Autodesk Fusion 360 part; units mm, degrees
(part 2 of 2)
sketch "Sketch21 (3)" plane through (0, 0, 1) normal (0, 0, 1) x (-1, 0, 0) in component "2"
  circle A0 centre (-8.5, 0) radius 9.5
  arc A1 (-18.8, -6.8) -> (-15.3, -10.3) centre (-15.3, -6.8) ccw
  line L0 (-18.8, -6.8) -> (-18.8, 6.8)
  arc A2 (-15.3, 10.3) -> (-18.8, 6.8) centre (-15.3, 6.8) ccw
  line L1 (-15.3, 10.3) -> (21, 10.3)
  line L2 (21, 10.3) -> (21, -10.3)
  line L3 (21, -10.3) -> (-15.3, -10.3)
  line L4 (1.8, -10.3) -> (1.8, 10.3)
  line L5 (0, 0) -> (-18.8, 0) construction
  arc A3 (-21, -7.5) -> (-17.5, -11) centre (-17.5, -7.5) ccw
  line L6 (-17.5, -11) -> (17.5, -11)
  arc A4 (17.5, -11) -> (21, -7.5) centre (17.5, -7.5) ccw
  line L7 (21, -7.5) -> (21, 7.5)
  arc A5 (21, 7.5) -> (17.5, 11) centre (17.5, 7.5) ccw
  line L8 (17.5, 11) -> (-17.5, 11)
  arc A6 (-17.5, 11) -> (-21, 7.5) centre (-17.5, 7.5) ccw
  line L9 (-21, 7.5) -> (-21, -7.5)
  circle A7 centre (-8, 0) radius 6.5
  circle A8 centre (12.6, 0) radius 6.5
  dimension "d400_1" = 19
  dimension "d401_1" = 20.6
  constraint coincident L3 L4.start
  constraint coincident L1 L4.end
  constraint perpendicular L1 L4
  constraint coincident L5.start origin
  constraint midpoint L0 L5.end
  constraint coincident A0.centre L5
  measures "d400_1" diameter of A0
  measures "d401_1" distance of L0 L4
fillet "Fillet10'" radius 3.5 8 edges at (21, -11, 0) (21, 11, 0) (-21, 11, 0) (-21, -11, 0) (19, -9, 1) (19, 9, 1) (-19, 9, 1) (-19, -9, 1) on bodies 2 in component "1"
sketch "Sketch18 (4)" plane through (-21, 0, 0) normal (-1, 0, 0) x (0, -1, 0) in component "1"
  line L0 (7.5, -3) -> (7.5, 3)
  line L1 (7.5, 3) -> (-7.5, 3)
  line L2 (-7.5, 3) -> (-7.5, -3)
  line L3 (-7.5, -3) -> (7.5, -3)
  line L4 (6, 3) -> (-6, 3)
  line L5 (-6, 3) -> (-6, 0)
  line L6 (-6, 0) -> (6, 0)
  line L7 (6, 0) -> (6, 3)
  line L8 (6, 3) -> (-6, 0) construction
  line L9 (-6, 3) -> (6, 0) construction
  line L10 (0, -3) -> (0, 3)
  point P0 (0, 1.5)
  dimension "d458" = 12
  dimension "d459" = 3
  constraint horizontal L4
  constraint perpendicular L4 L5
  constraint parallel L4 L6
  constraint parallel L5 L7
  constraint coincident L1 L4.start
  constraint coincident L8 P0
  constraint coincident L9 P0
  constraint midpoint L3 L10.start
  constraint midpoint L4 L10.end
  constraint vertical L10
  measures "d458" distance of L5.end L6.end
  measures "d459" distance of L4.start L6.end
extrude "Extrude17'" cut sketch "Sketch18 (4)" against normal blind 2.7 contours L1 L4 L6 L7 L10 | L1 L4 L5 L6 L10 bodies 2 in component "1"
sketch "Sketch19" plane through (0, 11, 0) normal (0, 1, 0) x (-1, 0, 0) in component "1"
  line L0 (17.5, -3) -> (17.5, 3)
  line L1 (17.5, 3) -> (-17.5, 3)
  line L2 (-17.5, 3) -> (-17.5, -3)
  line L3 (-17.5, -3) -> (17.5, -3)
  line L4 (-17.5, 0) -> (-16.9461, 0)
  line L5 (-16.9461, 0) -> (17.5, 0)
  point P0 (-12, 0)
  point P1 (12, 0)
  dimension "d462" = 12
  dimension "d463" = 12
  constraint midpoint L2 L4.start
  constraint perpendicular L2 L4
  constraint midpoint L0 L5.end
  constraint perpendicular L0 L5
  constraint coincident L5 P0
  constraint coincident L5 P1
  measures "d462" distance of origin P0
  measures "d463" distance of origin P1
hole "Hole2'" at (12, 11, 0) at (-12, 11, 0) direction (0, -1, 0) diameter 2.529 depth 2 tip angle 118 bodies 2 in component "1"
thread "Thread1" "ISO Metric profile 3.0 M3x0.5 6H" in component "1"
mirror "Mirror1" about plane through (0, 0, 0) normal (0, 1, 0) of "Hole2'" in component "1"
sketch "Sketch1 (10)" plane through (0, 0, 0) normal (0, 0, 1) x (1, 0, 0) in component "Resistance Paer"
  line L0 (17, 9) -> (-17, 9)
  line L1 (-17, 9) -> (-17, -9)
  line L2 (-17, -9) -> (17, -9)
  line L3 (17, -9) -> (17, 9)
  line L4 (17, 9) -> (-17, -9) construction
  line L5 (-17, 9) -> (17, -9) construction
  dimension "d138_1" = 18
  dimension "d139_1" = 34
  constraint horizontal L0
  constraint perpendicular L0 L1
  constraint parallel L0 L2
  constraint parallel L1 L3
  constraint coincident L4 origin
  constraint coincident L5 origin
  measures "d138_1" distance of L0.start L2.end
  measures "d139_1" distance of L0.start L0.end
extrude "Extrude1''''''''''''''" add sketch "Sketch1 (10)" along normal blind 0.06 separate body makes body 17 in component "Resistance Paer"
sketch "Sketch1 (11)" plane through (0, 0, 0) normal (0, 0, -1) x (1, 0, 0) in component "nylon wire vertical"
  line L0 (17, -9) -> (17, 9) construction
  line L1 (17, 9) -> (-17, 9) construction
  line L2 (-17, 9) -> (-17, -9)
  line L3 (-17, -9) -> (17, -9) construction
  line L4 (15, 8) -> (-15, 8) construction
  line L5 (-15, 8) -> (-15, -8) construction
  line L6 (-15, -8) -> (15, -8) construction
  line L7 (15, -8) -> (15, 8) construction
  line L8 (15, 8) -> (-15, -8) construction
  line L9 (-15, 8) -> (15, -8) construction
  line L10 (15, 8) -> (-15, 8)
  line L11 (-15, 8) -> (-15, 3)
  line L12 (-15, 3) -> (15, 3)
  line L13 (15, 3) -> (15, 8)
  line L14 (15, 8) -> (-15, 3) construction
  line L15 (-15, 8) -> (15, 3) construction
  line L16 (15, -8) -> (-15, -8)
  line L17 (-15, -8) -> (-15, -3)
  line L18 (-15, -3) -> (15, -3)
  line L19 (15, -3) -> (15, -8)
  line L20 (15, -8) -> (-15, -3) construction
  line L21 (-15, -8) -> (15, -3) construction
  point P0 (0, 5.5)
  point P1 (0, -5.5)
  dimension "d151_1" = 5
  dimension "d153_1" = 2
  dimension "d172_1" = 6
  constraint horizontal L4
  constraint perpendicular L4 L5
  constraint parallel L4 L6
  constraint parallel L5 L7
  constraint coincident L8 origin
  constraint coincident L9 origin
  constraint horizontal L10
  constraint perpendicular L10 L11
  constraint parallel L10 L12
  constraint parallel L11 L13
  constraint coincident L14 P0
  constraint coincident L15 P0
  constraint horizontal L16
  constraint perpendicular L16 L17
  constraint parallel L16 L18
  constraint parallel L17 L19
  constraint coincident L20 P1
  constraint coincident L21 P1
  constraint equal L11 L17
  constraint coincident L5 L11.end
  measures "d151_1" distance of L4.end L11.end
  measures "d153_1" distance of L2 L5
  measures "d172_1" distance of L12 L18
extrude "Extrude1'''''''''''''''" add sketch "Sketch1 (11)" along normal blind 0.2 separate body makes body 18 at (5, -4.6667, 0) makes body 19 at (5, 4.6667, 0) in component "nylon wire vertical"
move_face "OffsetFaces1" offset 3 2 faces at (15, 6.3333, -0.1333) (15, -6.3333, -0.1333) on bodies 18 19 in component "nylon wire vertical"
sketch "Sketch2 (4)" plane through (0, 0, 0) normal (0, 0, 1) x (-1, 0, 0) in component "nylon wire vertical"
  line L0 (-18, 8) -> (-18, 3)
  line L1 (-18, 3) -> (15, 3)
  line L2 (15, 3) -> (15, 8)
  line L3 (15, 8) -> (-18, 8)
  line L4 (-18, -8) -> (-17.8, -8)
  line L5 (-17.8, -8) -> (-17.8, -3)
  line L6 (-17.8, -3) -> (-18, -3)
  line L7 (-18, -3) -> (-18, -8)
  line L8 (-18, -8) -> (-17.8, -3) construction
  line L9 (-17.8, -8) -> (-18, -3) construction
  line L10 (-18, 3) -> (-17.8, 3)
  line L11 (-17.8, 3) -> (-17.8, 8)
  line L12 (-17.8, 8) -> (-18, 8)
  line L13 (-18, 8) -> (-18, 3)
  line L14 (-18, 3) -> (-17.8, 8) construction
  line L15 (-17.8, 3) -> (-18, 8) construction
  point P0 (-17.9, -5.5)
  point P1 (-17.9, 5.5)
  point P2 (-18, -8)
  point P3 (-18, -3)
  dimension "d157_1" = 0.2
  constraint horizontal L4
  constraint perpendicular L4 L5
  constraint parallel L4 L6
  constraint parallel L5 L7
  constraint coincident L8 P0
  constraint coincident L9 P0
  constraint horizontal L10
  constraint perpendicular L10 L11
  constraint parallel L10 L12
  constraint parallel L11 L13
  constraint coincident L0.end L1.start
  constraint coincident L14 P1
  constraint coincident L15 P1
  constraint coincident P2 L4.start
  constraint coincident P3 L6.end
  constraint coincident L0.start L3.end
  constraint equal L6 L10
  measures "d157_1" distance of L11.end L0.start
extrude "Extrude2''''" add sketch "Sketch2 (4)" along normal blind 8 contours L0 L1 L3 L10 L11 L12 L13 | L4 L5 L6 L7 bodies 18 19 in component "nylon wire vertical"
sketch "Sketch1 (12)" plane through (0, 0, 0) normal (0, 0, -1) x (1, 0, 0) in component "termistor (2)"
  line L0 (17, -9) -> (17, 9)
  line L1 (17, 9) -> (-17, 9)
  line L2 (-17, 9) -> (-17, -9)
  line L3 (-17, -9) -> (17, -9)
  line L4 (-2.5, 2.5) -> (18, 2.5)
  line L5 (18, 2.5) -> (18, -2.5)
  line L6 (18, -2.5) -> (-2.5, -2.5)
  line L7 (-2.5, -2.5) -> (-2.5, 2.5)
  line L8 (-2.5, 2.5) -> (18, -2.5) construction
  line L9 (18, 2.5) -> (-2.5, -2.5) construction
  line L10 (18, 3) -> (18, 8)
  line L11 (0, 0) -> (7.75, 0) construction
  line L12 (-2.5, -8) -> (-2.5, 8)
  point P0 (7.75, 0)
  dimension "d160_2" = 5
  constraint horizontal L4
  constraint perpendicular L4 L5
  constraint parallel L4 L6
  constraint parallel L5 L7
  constraint coincident L8 P0
  constraint coincident L9 P0
  constraint coincident L4.end L10
  constraint coincident L11.start origin
  constraint horizontal L11
  constraint coincident P0 L11.end
  constraint coincident L4.start L12
  measures "d160_2" distance of L4.start L6.end
extrude "Extrude1''''''''''''''''" add sketch "Sketch1 (12)" along normal blind 0.2 separate body contours L0 L4 L6 L7 L12 | L0 L4 L5 L6 makes body 20 in component "termistor (2)"
sketch "Sketch2 (5)" plane through (0, 0, 0) normal (0, 0, 1) x (-1, 0, 0) in component "termistor (2)"
  line L0 (-18, 2.5) -> (-18, -2.5)
  line L1 (-18, -2.5) -> (2.5, -2.5)
  line L2 (2.5, -2.5) -> (2.5, 2.5)
  line L3 (2.5, 2.5) -> (-18, 2.5)
  line L4 (-18, -2.5) -> (-17.8, -2.5)
  line L5 (-17.8, -2.5) -> (-17.8, 2.5)
  line L6 (-17.8, 2.5) -> (-18, 2.5)
  line L7 (-18, 2.5) -> (-18, -2.5)
  line L8 (-18, -2.5) -> (-17.8, 2.5) construction
  line L9 (-17.8, -2.5) -> (-18, 2.5) construction
  line L10 (-18, -0.9562) -> (-17.8, -0.9562)
  line L11 (-17.8, -0.9562) -> (-17.8, 0.9562)
  line L12 (-17.8, 0.9562) -> (-18, 0.9562)
  line L13 (-18, 0.9562) -> (-18, -0.9562)
  line L14 (-18, -0.9562) -> (-17.8, 0.9562) construction
  line L15 (-17.8, -0.9562) -> (-18, 0.9562) construction
  point P0 (-17.9, 0)
  point P1 (-17.9, 0)
  dimension "d163_2" = 0.2
  constraint horizontal L4
  constraint perpendicular L4 L5
  constraint parallel L4 L6
  constraint parallel L5 L7
  constraint coincident L0.end L1.start
  constraint coincident L8 P1
  constraint coincident L9 P1
  constraint coincident L0.start L3.end
  constraint horizontal L10
  constraint perpendicular L10 L11
  constraint parallel L10 L12
  constraint parallel L11 L13
  constraint coincident L7 L10.start
  constraint coincident L14 P1
  constraint coincident L15 P1
  constraint coincident P1 P0
  measures "d163_2" distance of L5.end L0.start
extrude "Extrude2'''''" add sketch "Sketch2 (5)" along normal blind 7 contours L0 L3 L5 L6 L7 L12 | L0 L1 L4 L5 L7 L10 bodies 20 in component "termistor (2)"
sketch "Sketch1 (13)" plane through (0, 0, 0) normal (0, 0, 1) x (1, 0, 0) in component "silicon membrane"
  line L0 (19, 10.5) -> (-19, 10.5)
  line L1 (-19, 10.5) -> (-19, -10.5)
  line L2 (-19, -10.5) -> (19, -10.5)
  line L3 (19, -10.5) -> (19, 10.5)
  line L4 (19, 10.5) -> (-19, -10.5) construction
  line L5 (-19, 10.5) -> (19, -10.5) construction
  dimension "d166_1" = 21
  dimension "d167_1" = 38
  constraint horizontal L0
  constraint perpendicular L0 L1
  constraint parallel L0 L2
  constraint parallel L1 L3
  constraint coincident L4 origin
  constraint coincident L5 origin
  measures "d166_1" distance of L0.start L2.end
  measures "d167_1" distance of L0.start L0.end
extrude "Extrude1'''''''''''''''''" add sketch "Sketch1 (13)" along normal mid plane 3.5 separate body makes body 21 in component "silicon membrane"
fillet "Fillet1" radius 3.5 4 edges at (-19, 10.5, 0) (-19, -10.5, 0) (19, -10.5, 0) (19, 10.5, 0) on bodies 21 in component "silicon membrane"
sketch "Sketch4 (2)" plane through (0, 0, 1.75) normal (0, 0, 1) x (-1, 0, 0) in component "Silicon Tactile  (2)"
  arc A0 (-19, -7) -> (-15.5, -10.5) centre (-15.5, -7) ccw
  line L0 (-15.5, -10.5) -> (15.5, -10.5)
  arc A1 (15.5, -10.5) -> (19, -7) centre (15.5, -7) ccw
  line L1 (19, -7) -> (19, 7)
  arc A2 (19, 7) -> (15.5, 10.5) centre (15.5, 7) ccw
  line L2 (15.5, 10.5) -> (-15.5, 10.5)
  arc A3 (-15.5, 10.5) -> (-19, 7) centre (-15.5, 7) ccw
  line L3 (-19, 7) -> (-19, -7)
  line L4 (0, 0) -> (0, 7.8)
  line L5 (0, 0) -> (-17.8, 0)
  line L6 (-18, 8) -> (-18, 3)
  line L7 (-18, 3) -> (-17.8, 3)
  line L8 (-17.8, 3) -> (-17.8, 8)
  line L9 (-17.8, 8) -> (-18, 8)
  line L10 (-17.8, 2.5) -> (-18, 2.5)
  line L11 (-18, 2.5) -> (-18, 0.9562)
  line L12 (-18, 0.9562) -> (-17.8, 0.9562)
  line L13 (-17.8, 0.9562) -> (-17.8, 2.5)
  line L14 (-18, -2.5) -> (-17.8, -2.5)
  line L15 (-17.8, -2.5) -> (-17.8, -0.9562)
  line L16 (-17.8, -0.9562) -> (-18, -0.9562)
  line L17 (-18, -0.9562) -> (-18, -2.5)
  line L18 (-18, -3) -> (-18, -8)
  line L19 (-18, -8) -> (-17.8, -8)
  line L20 (-17.8, -8) -> (-17.8, -3)
  line L21 (-17.8, -3) -> (-18, -3)
  line L22 (-13.5, 7.8) -> (-8.5, 7.8)
  line L23 (-8.5, 7.8) -> (-8.5, 8)
  line L24 (-8.5, 8) -> (-13.5, 8)
  line L25 (-13.5, 8) -> (-13.5, 7.8)
  line L26 (-2.5, 7.8) -> (2.5, 7.8)
  line L27 (2.5, 7.8) -> (2.5, 8)
  line L28 (2.5, 8) -> (-2.5, 8)
  line L29 (-2.5, 8) -> (-2.5, 7.8)
  line L30 (8.5, 7.8) -> (13.5, 7.8)
  line L31 (13.5, 7.8) -> (13.5, 8)
  line L32 (13.5, 8) -> (8.5, 8)
  line L33 (8.5, 8) -> (8.5, 7.8)
  line L34 (13.65, 8.15) -> (8.35, 8.15)
  line L35 (8.35, 8.15) -> (8.35, 7.65)
  line L36 (8.35, 7.65) -> (13.65, 7.65)
  line L37 (13.65, 7.65) -> (13.65, 8.15)
  line L38 (2.65, 8.15) -> (-2.65, 8.15)
  line L39 (-2.65, 8.15) -> (-2.65, 7.65)
  line L40 (-2.65, 7.65) -> (2.65, 7.65)
  line L41 (2.65, 7.65) -> (2.65, 8.15)
  line L42 (-8.35, 8.15) -> (-13.65, 8.15)
  line L43 (-13.65, 8.15) -> (-13.65, 7.65)
  line L44 (-13.65, 7.65) -> (-8.35, 7.65)
  line L45 (-8.35, 7.65) -> (-8.35, 8.15)
  line L46 (-18.15, 8.15) -> (-18.15, 2.85)
  line L47 (-18.15, 2.85) -> (-17.65, 2.85)
  line L48 (-17.65, 2.85) -> (-17.65, 8.15)
  line L49 (-17.65, 8.15) -> (-18.15, 8.15)
  line L50 (-18.15, 2.65) -> (-18.15, 0.8062)
  line L51 (-18.15, 0.8062) -> (-17.65, 0.8062)
  line L52 (-17.65, 0.8062) -> (-17.65, 2.65)
  line L53 (-17.65, 2.65) -> (-18.15, 2.65)
  line L54 (-18.15, -0.8062) -> (-18.15, -2.65)
  line L55 (-18.15, -2.65) -> (-17.65, -2.65)
  line L56 (-17.65, -2.65) -> (-17.65, -0.8062)
  line L57 (-17.65, -0.8062) -> (-18.15, -0.8062)
  line L58 (-18.15, -2.85) -> (-18.15, -8.15)
  line L59 (-18.15, -8.15) -> (-17.65, -8.15)
  line L60 (-17.65, -8.15) -> (-17.65, -2.85)
  line L61 (-17.65, -2.85) -> (-18.15, -2.85)
  dimension "d177_1" = 0.15
  dimension "d178_1" = 0.15
  dimension "d179_1" = 0.15
  dimension "d180_1" = 0.15
  dimension "d181_1" = 0.15
  dimension "d182_1" = 0.15
  dimension "d183_1" = 0.15
  constraint coincident L4.start L5.start
  constraint vertical L4
  constraint perpendicular L4 L5
  constraint midpoint L4.end L26
  constraint coincident L5.end L15
sketch "Sketch17 (3)" plane through (0, 0, 0) normal (0, 0, 1) x (1, 0, 0) in component "4"
  line L0 (21.5, 11.5) -> (-21.5, 11.5)
  line L1 (-21.5, 11.5) -> (-21.5, -11.5)
  line L2 (-21.5, -11.5) -> (21.5, -11.5)
  line L3 (21.5, -11.5) -> (21.5, 11.5)
  line L4 (21.5, 11.5) -> (-21.5, -11.5) construction
  line L5 (-21.5, 11.5) -> (21.5, -11.5) construction
  line L6 (-23.75, -13.75) -> (23.75, -13.75)
  line L7 (23.75, -13.75) -> (23.75, 13.75)
  line L8 (23.75, 13.75) -> (-23.75, 13.75)
  line L9 (-23.75, 13.75) -> (-23.75, -13.75)
  dimension "d1_1_1_1" = 43
  dimension "d2_1_1_1" = 23
  dimension "d3_1_1_1" = 2.25
  constraint horizontal L0
  constraint perpendicular L0 L1
  constraint parallel L0 L2
  constraint parallel L1 L3
  constraint coincident L4 origin
  constraint coincident L5 origin
  measures "d1_1_1_1" distance of L0.start L0.end
  measures "d2_1_1_1" distance of L0.start L2.end
extrude "Extrude17''" add sketch "Sketch17 (3)" against normal blind 14 separate body makes body 22 in component "4"
sketch "Sketch29" plane through (0, 0, 1) normal (0, 0, 1) x (-1, 0, 0) in component "2"
  circle A0 centre (12.6, 0) radius 3.5
  circle A1 centre (12.6, 0) radius 4.5
sketch "Sketch30" plane through (21, 0, 0) normal (1, 0, 0) x (0, 1, 0) in component "2"
  line L0 (7.5, -1) -> (7.5, 1)
  line L1 (7.5, 1) -> (-7.5, 1)
  line L2 (-7.5, 1) -> (-7.5, -1)
  line L3 (-7.5, -1) -> (7.5, -1)
  line L4 (0, 0) -> (0, -1)
  line L5 (6, -1) -> (-6, -1)
  line L6 (-6, -1) -> (-6, 1.5539)
  line L7 (-6, 1.5539) -> (6, 1.5539)
  line L8 (6, 1.5539) -> (6, -1)
  line L9 (6, -1) -> (-6, 1.5539) construction
  line L10 (-6, -1) -> (6, 1.5539) construction
  point P0 (0, 0.277)
  dimension "d485" = 12
  constraint coincident L4.start origin
  constraint midpoint L3 L4.end
  constraint horizontal L5
  constraint perpendicular L5 L6
  constraint parallel L5 L7
  constraint parallel L6 L8
  constraint coincident L3 L5.start
  constraint coincident L9 P0
  constraint coincident L10 P0
  constraint coincident L4 P0
  measures "d485" distance of L6.end L7.end
extrude "Extrude34" cut sketch "Sketch30" against normal blind 7 contours L1 L3 L5 L6 L8 | L1 L6 L7 L8 bodies 16 in component "2"
sketch "Sketch18 (5)" plane through (0, 0, -3) normal (0, 0, -1) x (1, 0, 0) in component "3"
  arc A0 (-17.5, 11) -> (-21, 7.5) centre (-17.5, 7.5) ccw
  line L0 (-21, 7.5) -> (-21, -7.5)
  arc A1 (-21, -7.5) -> (-17.5, -11) centre (-17.5, -7.5) ccw
  line L1 (-17.5, -11) -> (17.5, -11)
  arc A2 (17.5, -11) -> (21, -7.5) centre (17.5, -7.5) ccw
  line L2 (21, -7.5) -> (21, 7.5)
  arc A3 (21, 7.5) -> (17.5, 11) centre (17.5, 7.5) ccw
  line L3 (17.5, 11) -> (-17.5, 11) construction
  line L4 (-21, 0) -> (21, 0) construction
  circle A4 centre (-12.6, 0) radius 5.5 construction
  circle A5 centre (12.6, 0) radius 5.5 construction
  circle A6 centre (-12.6, 0) radius 6.5
  circle A7 centre (-12.6, 0) radius 4.5
  circle A8 centre (12.6, 0) radius 6.5
  circle A9 centre (12.6, 0) radius 4
  line L5 (-15, 5) -> (-15, -5)
  line L6 (-15, -5) -> (-19, -5)
  line L7 (-19, -5) -> (-19, 5)
  line L8 (-19, 5) -> (-15, 5)
  dimension "d491" = 11
  dimension "d492" = 8.4
  dimension "d493" = 8.4
  dimension "d494" = 1
  dimension "d495" = -1
  dimension "d496" = 1
  dimension "d497" = -1.5
  constraint midpoint L0 L4.start
  constraint midpoint L2 L4.end
  constraint coincident L4 A4.centre
  constraint coincident L4 A5.centre
  constraint equal A4 A5
  measures "d491" diameter of A4
  measures "d492" distance of L4.start A4.centre
  measures "d493" distance of L4.end A5.centre
extrude "Extrude19" cut sketch "Sketch18 (5)" against normal blind 2 contours A6 A7 L5 L6 L8 | A6 A7 L5 L6 L7 L8 | A6 L7 | A8 bodies 15 in component "3"
sketch "Sketch19 (2)" plane through (0, 0, -3) normal (0, 0, -1) x (1, 0, 0) in component "3"
  circle A0 centre (12.6, 0) radius 4
  circle A1 centre (12.6, 0) radius 2.75
  dimension "d500" = 5.5
  constraint concentric A0 A1
  measures "d500" diameter of A1
fillet "Fillet13" radius 3.5 8 edges at (21.5, 11.5, -7) (-21.5, 11.5, -7) (-21.5, -11.5, -7) (21.5, -11.5, -7) (-23.75, 13.75, -7) (23.75, 13.75, -7) (23.75, -13.75, -7) (-23.75, -13.75, -7) on bodies 22 in component "4"
sketch "Sketch19 (3)" plane through (0, -13.75, 0) normal (0, -1, 0) x (1, 0, 0) in component "4"
  line L0 (-20.25, 0) -> (-20.25, -14)
  line L1 (-20.25, -14) -> (20.25, -14)
  line L2 (20.25, -14) -> (20.25, 0)
  line L3 (20.25, 0) -> (-20.25, 0)
  line L4 (-20.25, -3) -> (20.25, -3)
  line L5 (-20.25, -11) -> (20.25, -11)
  point P0 (-12, -3)
  point P1 (12, -3)
  point P2 (-12, -11)
  point P3 (12, -11)
  dimension "d505" = 12
  dimension "d506" = 3
  dimension "d507" = 3
  dimension "d508" = 12
  dimension "d509" = 12
  dimension "d510" = 12
  constraint coincident L0 L4.start
  constraint coincident L2 L4.end
  constraint perpendicular L2 L4
  constraint coincident L4 P0
  constraint coincident L4 P1
  constraint coincident L0 L5.start
  constraint coincident L2 L5.end
  constraint perpendicular L2 L5
  constraint coincident L5 P2
  constraint coincident L5 P3
  measures "d505" horizontal distance of origin P0
  measures "d506" distance of L3 L4
  measures "d507" distance of L1 L5
  measures "d508" horizontal distance of origin P2
  measures "d509" horizontal distance of origin P3
  measures "d510" horizontal distance of origin P1
hole "Hole1" at (-12, -13.75, -3) at (-12, -13.75, -11) at (12, -13.75, -3) at (12, -13.75, -11) direction (0, 1, 0) diameter 2.529 depth 45 tip angle 118 bodies 22 in component "4"
thread "Thread1'" "ISO Metric profile 3.0 M3x0.5 6H" in component "4"
sketch "Sketch20 (4)" plane through (0, 13.75, 0) normal (0, 1, 0) x (-1, 0, 0) in component "4"
  circle A0 centre (-12, -3) radius 1.2645
  circle A1 centre (12, -3) radius 1.2645
  circle A2 centre (12, -11) radius 1.2645
  circle A3 centre (-12, -11) radius 1.2645
  line L0 (-20.25, 0) -> (-20.25, -14)
  line L1 (-20.25, -14) -> (20.25, -14)
  line L2 (20.25, -14) -> (20.25, 0)
  line L3 (20.25, 0) -> (-20.25, 0)
  line L4 (-3, -11) -> (-3, -3)
  arc A4 (-3, -3) -> (-5, -3) centre (-4, -3) ccw
  line L5 (-5, -3) -> (-5, -11)
  arc A5 (-5, -11) -> (-3, -11) centre (-4, -11) ccw
  line L6 (-4, -11) -> (-4, -3) construction
  line L7 (0, 0) -> (0, -14) construction
  line L8 (4, 0) -> (4, -14) construction
  line L9 (-4, -14) -> (-4, 0) construction
  line L10 (3, -11) -> (3, -3)
  line L11 (5, -3) -> (5, -11)
  arc A6 (5, -3) -> (3, -3) centre (4, -3) ccw
  arc A7 (3, -11) -> (5, -11) centre (4, -11) ccw
  point P0 (-4, -7)
  dimension "d524" = 2
  dimension "d525" = 8
  dimension "d562" = 4
  dimension "d564" = 4
  dimension "d565" = 3
  constraint tangent L4 A4
  constraint tangent A4 L5
  constraint parallel L4 L5
  constraint tangent L5 A5
  constraint tangent L4 A5
  constraint coincident L6 P0
  constraint midpoint L6 P0
  constraint coincident L7.start origin
  constraint midpoint L1 L7.end
  constraint coincident L3 L8.start
  constraint coincident L1 L8.end
  constraint perpendicular L1 L8
  constraint coincident L1 L9.start
  constraint coincident L3 L9.end
  constraint perpendicular L3 L9
  constraint coincident P0 L9
  constraint coincident A4.centre L9
  constraint symmetric L4.start L7 L10.start
  constraint symmetric L4.end L7 L10.end
  constraint symmetric A4.end L7 L11.start
  constraint symmetric L5.end L7 L11.end
  constraint symmetric A4 L7 A6
  constraint symmetric A5 L7 A7
  measures "d524" distance of L4 L5
  measures "d525" distance of A4.end L5.end
  measures "d562" distance of A4.centre L7
  measures "d564" distance of L7 L8
  measures "d565" distance of L3 A6.centre
extrude "Extrude21" cut sketch "Sketch20 (4)" against normal blind 27.5 contours L4 A4 L5 A5 | L10 L11 A6 A7 bodies 22 in component "4"
sketch "Sketch31" plane through (0, 0, 1) normal (0, 0, 1) x (-1, 0, 0) in component "2"
  line L0 (-14, -6) -> (-21, -6)
  line L1 (-21, -6) -> (-21, -7.5)
  arc A0 (-21, -7.5) -> (-17.5, -11) centre (-17.5, -7.5) ccw
  line L2 (-17.5, -11) -> (17.5, -11)
  arc A1 (17.5, -11) -> (21, -7.5) centre (17.5, -7.5) ccw
  line L3 (21, -7.5) -> (21, 7.5)
  arc A2 (21, 7.5) -> (17.5, 11) centre (17.5, 7.5) ccw
  line L4 (17.5, 11) -> (-17.5, 11)
  arc A3 (-17.5, 11) -> (-21, 7.5) centre (-17.5, 7.5) ccw
  line L5 (-21, 7.5) -> (-21, 6)
  line L6 (-21, 6) -> (-14, 6)
  arc A4 (-14, -2.5) -> (-14, 2.5) centre (-8, 0) ccw
  circle A5 centre (12.6, 0) radius 6.5
  spline S0 degree 5 poles (0, -11) (0, -10.12) (0, -8.36) (0, -5.72) (0, -2.2) (0, 2.2) (0, 5.72) (0, 8.36) (0, 10.12) (0, 11) knots 0 0 0 0 0 0 0.2 0.4 0.6 0.8 1 1 1 1 1 1
  line L7 (-7.5, -8) -> (7.5, -8)
  line L8 (7.5, -8) -> (7.5, -14)
  line L9 (7.5, -14) -> (-7.5, -14)
  line L10 (-7.5, -14) -> (-7.5, -8)
  line L11 (-7.5, -8) -> (7.5, -14) construction
  line L12 (7.5, -8) -> (-7.5, -14) construction
  line L13 (-7.5, 8) -> (7.5, 8)
  line L14 (7.5, 8) -> (7.5, 14)
  line L15 (7.5, 14) -> (-7.5, 14)
  line L16 (-7.5, 14) -> (-7.5, 8)
  line L17 (-7.5, 8) -> (7.5, 14) construction
  line L18 (7.5, 8) -> (-7.5, 14) construction
  line L19 (-14, 6) -> (-14, 2.5)
  line L20 (-14, -2.5) -> (-14, -6)
  point P0 (0, -11)
  point P1 (0, 11)
  dimension "d528" = 6
  dimension "d529" = 6
  dimension "d530" = 15
  dimension "d531" = 15
  constraint midpoint L2 P0
  constraint midpoint L4 P1
  constraint horizontal L7
  constraint perpendicular L7 L8
  constraint parallel L7 L9
  constraint parallel L8 L10
  constraint coincident L11 P0
  constraint coincident L12 P0
  constraint coincident P0 S0.start
  constraint horizontal L13
  constraint perpendicular L13 L14
  constraint parallel L13 L15
  constraint parallel L14 L16
  constraint coincident L17 P1
  constraint coincident L18 P1
  constraint coincident P1 S0.end
  measures "d528" distance of L13.start L15.end
  measures "d529" distance of L7.start L9.end
  measures "d530" distance of L8.end L9.end
  measures "d531" distance of L13.start L13.end
extrude "Extrude35" cut sketch "Sketch31" against normal blind 2 contours L2 S0 L7 L10 | L2 S0 L7 L8 | L4 S0 L13 L16 | L4 S0 L13 L14 bodies 16 in component "2"
sketch "Sketch20 (5)" plane through (0, 0, 3) normal (0, 0, 1) x (-1, 0, 0) in component "1"
  line L0 (21, -6) -> (18.9641, -6)
  arc A0 (15.5, -9) -> (18.9641, -6) centre (15.5, -5.5) ccw
  line L1 (15.5, -9) -> (-15.5, -9)
  arc A1 (-19, -5.5) -> (-15.5, -9) centre (-15.5, -5.5) ccw
  line L2 (-19, -5.5) -> (-19, 5.5)
  arc A2 (-15.5, 9) -> (-19, 5.5) centre (-15.5, 5.5) ccw
  line L3 (-15.5, 9) -> (15.5, 9)
  arc A3 (18.9641, 6) -> (15.5, 9) centre (15.5, 5.5) ccw
  line L4 (18.9641, 6) -> (21, 6)
  line L5 (21, 6) -> (21, 7.5)
  arc A4 (21, 7.5) -> (17.5, 11) centre (17.5, 7.5) ccw
  line L6 (17.5, 11) -> (-17.5, 11)
  arc A5 (-17.5, 11) -> (-21, 7.5) centre (-17.5, 7.5) ccw
  line L7 (-21, 7.5) -> (-21, -7.5)
  arc A6 (-21, -7.5) -> (-17.5, -11) centre (-17.5, -7.5) ccw
  line L8 (-17.5, -11) -> (17.5, -11)
  arc A7 (17.5, -11) -> (21, -7.5) centre (17.5, -7.5) ccw
  line L9 (21, -7.5) -> (21, -6)
  line L10 (0, -11) -> (0, 11)
  line L11 (-7.5, -8) -> (7.5, -8)
  line L12 (7.5, -8) -> (7.5, -14)
  line L13 (7.5, -14) -> (-7.5, -14)
  line L14 (-7.5, -14) -> (-7.5, -8)
  line L15 (-7.5, -8) -> (7.5, -14) construction
  line L16 (7.5, -8) -> (-7.5, -14) construction
  line L17 (-7.5, 8) -> (7.5, 8)
  line L18 (7.5, 8) -> (7.5, 14)
  line L19 (7.5, 14) -> (-7.5, 14)
  line L20 (-7.5, 14) -> (-7.5, 8)
  line L21 (-7.5, 8) -> (7.5, 14) construction
  line L22 (7.5, 8) -> (-7.5, 14) construction
  point P0 (0, -11)
  point P1 (0, 11)
  dimension "d534" = 15
  dimension "d535" = 6
  dimension "d536" = 6
  dimension "d537" = 15
  constraint midpoint L8 P0
  constraint midpoint L6 P1
  constraint horizontal L11
  constraint perpendicular L11 L12
  constraint parallel L11 L13
  constraint parallel L12 L14
  constraint coincident L15 P0
  constraint coincident L16 P0
  constraint coincident P0 L10.start
  constraint horizontal L17
  constraint perpendicular L17 L18
  constraint parallel L17 L19
  constraint parallel L18 L20
  constraint coincident L21 P1
  constraint coincident L22 P1
  constraint coincident P1 L10.end
  measures "d534" distance of L12.end L13.end
  measures "d535" distance of L11.start L13.end
  measures "d536" distance of L17.start L19.end
  measures "d537" distance of L18.end L19.end
extrude "Extrude18''" cut sketch "Sketch20 (5)" against normal blind 6 contours L1 L8 L10 L12 | L1 L10 L11 L12 | L1 L8 L10 L14 | L1 L10 L11 L14 | L3 L10 L17 L20 | L3 L10 L17 L18 | L3 L6 L10 L18 | L3 L6 L10 L20 bodies 2 in component "1"
sketch "Sketch20 (6)" plane through (0, 0, -3) normal (0, 0, -1) x (1, 0, 0) in component "3"
  circle A0 centre (12.6, 0) radius 6.5
  arc A1 (-16.7533, -5) -> (-16.7533, 5) centre (-12.6, 0) ccw
  line L0 (-16.7533, -5) -> (-19, -5)
  line L1 (-19, -5) -> (-19, -1.1358)
  arc A2 (-19, 1.1358) -> (-19, -1.1358) centre (-12.6, 0) ccw
  line L2 (-19, 1.1358) -> (-19, 5)
  line L3 (-19, 5) -> (-16.7533, 5)
  arc A3 (-17.5, 11) -> (-21, 7.5) centre (-17.5, 7.5) ccw
  line L4 (-21, 7.5) -> (-21, -7.5)
  arc A4 (-21, -7.5) -> (-17.5, -11) centre (-17.5, -7.5) ccw
  line L5 (-17.5, -11) -> (17.5, -11)
  arc A5 (17.5, -11) -> (21, -7.5) centre (17.5, -7.5) ccw
  line L6 (21, -7.5) -> (21, 7.5)
  arc A6 (21, 7.5) -> (17.5, 11) centre (17.5, 7.5) ccw
  line L7 (17.5, 11) -> (-17.5, 11)
  spline S0 degree 5 poles (0, 11) (0, 10.12) (0, 8.36) (0, 5.72) (0, 2.2) (0, -2.2) (0, -5.72) (0, -8.36) (0, -10.12) (0, -11) knots 0 0 0 0 0 0 0.2 0.4 0.6 0.8 1 1 1 1 1 1
  line L8 (6, 11) -> (-6, 11)
  line L9 (-6, 11) -> (-6, 8.5)
  line L10 (-6, 8.5) -> (6, 8.5)
  line L11 (6, 8.5) -> (6, 11)
  line L12 (6, 11) -> (-6, 8.5) construction
  line L13 (-6, 11) -> (6, 8.5) construction
  line L14 (6, -11) -> (-6, -11)
  line L15 (-6, -11) -> (-6, -8.5)
  line L16 (-6, -8.5) -> (6, -8.5)
  line L17 (6, -8.5) -> (6, -11)
  line L18 (6, -11) -> (-6, -8.5) construction
  line L19 (-6, -11) -> (6, -8.5) construction
  point P0 (0, 9.75)
  point P1 (0, -9.75)
  dimension "d540" = 12
  dimension "d541" = 12
  dimension "d542" = 2.5
  dimension "d543" = 2.5
  constraint midpoint L7 S0.start
  constraint midpoint L5 S0.end
  constraint horizontal L8
  constraint perpendicular L8 L9
  constraint parallel L8 L10
  constraint parallel L9 L11
  constraint coincident L7 L8.start
  constraint coincident L12 P0
  constraint coincident L13 P0
  constraint coincident S0 P0
  constraint horizontal L14
  constraint perpendicular L14 L15
  constraint parallel L14 L16
  constraint parallel L15 L17
  constraint coincident L5 L14.start
  constraint coincident L18 P1
  constraint coincident L19 P1
  constraint coincident S0 P1
  measures "d540" distance of L9.end L10.end
  measures "d541" distance of L15.end L16.end
  measures "d542" distance of L14.start L16.end
  measures "d543" distance of L8.start L10.end
extrude "Extrude21'" add sketch "Sketch20 (6)" along normal blind 3 contours L7 S0 L8 L9 L10 | L7 S0 L8 L10 L11 | L5 S0 L14 L15 L16 | L5 S0 L14 L16 L17 bodies 15 in component "3"
sketch "Sketch21 (4)" plane through (0, -11, 0) normal (0, -1, 0) x (1, 0, 0) in component "3"
  line L0 (-17.5, 3) -> (-17.5, -3)
  line L1 (-17.5, -3) -> (-6, -3)
  line L2 (-6, -3) -> (-6, -6)
  line L3 (6, -6) -> (6, -3)
  line L4 (6, -3) -> (17.5, -3)
  line L5 (17.5, -3) -> (17.5, 3)
  line L6 (17.5, 3) -> (-17.5, 3)
  line L7 (6, -6) -> (6, -3)
  line L8 (-6, -3) -> (-6, -6)
  line L9 (0, 0) -> (0, -4.9341) construction
  line L10 (-4, -4) -> (4, -4)
  line L11 (6, -6) -> (-6, -6)
  point P0 (0, -4)
  dimension "d560" = 8
  dimension "d561" = 2
  constraint parallel L7 L8
  constraint coincident L3.start L7.start
  constraint coincident L2.end L8.end
  constraint coincident L4 L3.end
  constraint coincident L9.start origin
  constraint perpendicular L6 L9
  constraint horizontal L10
  constraint midpoint L10 P0
  constraint coincident L9 P0
  measures "d560" distance of L10.start L10.end
  measures "d561" distance of L10 L11
hole "Hole1'" at (-4, -11, -4) at (4, -11, -4) direction (0, 1, 0) diameter 2 depth 45 tip angle 118 bodies 15 in component "3"
sketch "Sketch21 (5)" plane through (-23.75, 0, 0) normal (-1, 0, 0) x (0, -1, 0) in component "4"
  line L0 (10.25, -14) -> (10.25, 0)
  line L1 (10.25, 0) -> (-10.25, 0)
  line L2 (-10.25, 0) -> (-10.25, -14)
  line L3 (-10.25, -14) -> (10.25, -14)
  line L4 (0, 0) -> (0, -14) construction
  line L5 (5.5, -12.5) -> (-5.5, -12.5)
  line L6 (-5.5, -12.5) -> (-5.5, -1.5)
  line L7 (-5.5, -1.5) -> (5.5, -1.5)
  line L8 (5.5, -1.5) -> (5.5, -12.5)
  line L9 (5.5, -12.5) -> (-5.5, -1.5) construction
  line L10 (-5.5, -12.5) -> (5.5, -1.5) construction
  point P0 (0, -7)
  dimension "d549" = 11
  dimension "d550" = 11
  constraint coincident L4.start origin
  constraint midpoint L3 L4.end
  constraint horizontal L5
  constraint perpendicular L5 L6
  constraint parallel L5 L7
  constraint parallel L6 L8
  constraint coincident L9 P0
  constraint coincident L10 P0
  constraint midpoint L4 P0
  measures "d549" distance of L5.start L7.end
  measures "d550" distance of L6.end L7.end
extrude "Extrude22" cut sketch "Sketch21 (5)" against normal blind 2.25 contours L5 L6 L7 L8 bodies 22 in component "4"
sketch "Sketch32" plane through (0, 0, 1) normal (0, 0, 1) x (-1, 0, 0) in component "2"
  circle A0 centre (12.6, 0) radius 4.5
  circle A1 centre (12.6, 0) radius 3.25
  dimension "d554" = 6.5
  constraint concentric A0 A1
  measures "d554" diameter of A1
extrude "Extrude36" cut sketch "Sketch32" against normal blind 2 contours A0 | A1 bodies 16 in component "2"
sketch "Sketch22 (2)" plane through (0, 0, -3) normal (0, 0, -1) x (1, 0, 0) in component "3"
  circle A0 centre (12.6, 0) radius 4
  circle A1 centre (12.6, 0) radius 2.75
  dimension "d557" = 5.5
  constraint coincident A0.centre A1.centre
  measures "d557" diameter of A1
extrude "Extrude22'" add sketch "Sketch22 (2)" along normal blind 3 bodies 15 in component "3"
component "1" placed x (1, 0, 0) y (0, 1, 0) z (0, 0, 1) at (0, 0, 0)
component "49E Hall Sensor LM393" placed x (1, 0, 0) y (0, 1, 0) z (0, 0, 1) at (-3.7, 0, -1)
component "cap 1" placed x (1, 0, 0) y (0, 1, 0) z (0, 0, 1) at (0, 1.5, 5)
component "Silicon Tactile " placed x (1, 0, 0) y (0, 1, 0) z (0, 0, 1) at (0, 0, 0)
component "FSR Load plate (1)" placed x (-1, 0, 0) y (0, -1, 0) z (0, 0, 1) at (8.5, 1.5, 78.1537)
component "cap 2" placed x (1, 0, 0) y (0, 1, 0) z (0, 0, 1) at (0, -1.5, 5)
component "Silicon Tactile  (1)" placed x (1, 0, 0) y (0, 1, 0) z (0, 0, 1) at (-2.0834, -0.2866, 15.927)
component "3" placed x (1, 0, 0) y (0, 1, 0) z (0, 0, 1) at (0, 0, 9.0324)
component "2" placed x (-1, 0, 0) y (0, -1, 0) z (0, 0, 1) at (0, 0, 4)
component "Silicon Tactile  (2)" placed x (-1, 0, 0) y (0, 1, 0) z (0, 0, -1) at (0, 0.25, 12.2824)
component "4" placed x (1, 0, 0) y (0, 1, 0) z (0, 0, 1) at (0, 0, 11)
component "FSR" placed x (1, 0, 0) y (0, 1, 0) z (0, 0, 1) at (8.5, 1.5, 84.1537) in component "Silicon Tactile "
component "termistor" placed x (-1, 0, 0) y (0, 1, 0) z (0, 0, -1) at (6, 1.5, 84.2137) in component "Silicon Tactile "
component "Foam" placed x (1, 0, 0) y (0, 1, 0) z (0, 0, 1) at (8.5, 1.5, 87.7137) in component "Silicon Tactile "
component "FSR (1)" placed x (1, 0, 0) y (0, 1, 0) z (0, 0, 1) at (6.9185, 14.0329, 47.5974) in component "Silicon Tactile  (1)"
component "termistor (1)" placed x (-1, 0, 0) y (0, 1, 0) z (0, 0, -1) at (4.4185, 14.0329, 47.6574) in component "Silicon Tactile  (1)"
component "Foam (1)" placed x (1, 0, 0) y (0, 1, 0) z (0, 0, 1) at (6.9185, 14.0329, 51.1574) in component "Silicon Tactile  (1)"
component "gen 2" placed x (1, 0, 0) y (0, 1, 0) z (0, 0, 1) at (10.175, 9.3282, 15.6109) in component "Silicon Tactile  (1)"
component "Resistance Paer" placed x (1, 0, 0) y (0, 1, 0) z (0, 0, 1) at (0, 0, 0) in component "Silicon Tactile  (2)"
component "nylon wire vertical" placed x (1, 0, 0) y (0, 1, 0) z (0, 0, 1) at (0, 0, 0) in component "Silicon Tactile  (2)"
component "termistor (2)" placed x (1, 0, 0) y (0, 1, 0) z (0, 0, 1) at (0, 0, 0) in component "Silicon Tactile  (2)"
component "silicon membrane" placed x (1, 0, 0) y (0, 1, 0) z (0, 0, 1) at (0, 0, 0) in component "Silicon Tactile  (2)"
equation "d287 = ( 11.6 / 2 ) * 1 mm"
equation "d6_1_1 = 3.5 mm - 1.5 mm"
